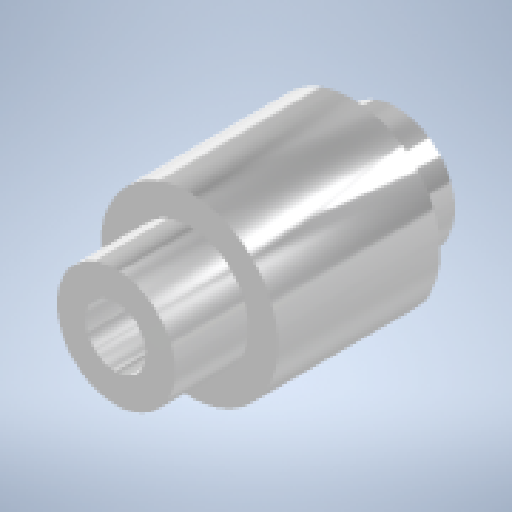
# Autodesk Inventor part: ベース板連結棒
Saved by Autodesk Inventor 2024 (Build 280153000, 153)
## iProperties
Created: 2023-05-30
Part Number: ベース板連結棒
Material: アルミニウム 6061
Document SubType Name: Modeling
Designer: yuta2
Density: 2.7 g/cm^3
Appearance: アルミニウム - フラット
Author: yuta2
Autodesk Inventor part; units mm, degrees
ref_plane "YZ Plane" through (0, 0, 0) normal (1, 0, 0) x (0, 1, 0)
ref_plane "XZ Plane" through (0, 0, 0) normal (0, 1, 0) x (-1, 0, 0)
ref_plane "XY Plane" through (0, 0, 0) normal (0, 0, 1) x (1, 0, 0)
sketch "スケッチ1" plane through (0, 0, 0) normal (1, 0, 0) x (0, 1, 0)
  line L0 (0, 0) -> (4, 0)
  line L1 (4, 0) -> (4, 5)
  line L2 (4, 5) -> (0, 5)
  line L3 (0, 5) -> (0, 0)
  line L4 (0, 0) -> (6, 0)
  line L5 (6, 0) -> (6, -11)
  line L6 (6, -11) -> (0, -11)
  line L7 (0, -11) -> (0, 0)
  line L8 (0, -11) -> (4, -11)
  line L9 (4, -11) -> (4, -14)
  line L10 (4, -14) -> (0, -14)
  line L11 (0, -14) -> (0, -11)
  dimension "d0" = 4
  dimension "d1" = 5
  dimension "d2" = 6
  dimension "d3" = 11
  dimension "d4" = 4
  dimension "d5" = 3
  constraints: 24 end point, 6 parallel, 3 horizontal, 3 perpendicular
  measures "d0" distance of L2.end L1.end
  measures "d1" distance of L1.end L0.end
  measures "d2" distance of L5.end L6.end
  measures "d3" distance of L4.end L5.end
  measures "d4" distance of L9.end L10.end
  measures "d5" distance of L8.end L9.end
revolve "回転1" add sketch "スケッチ1" angle 360 about axis through (0, 0, -11) along (0, 0, 1)
sketch "スケッチ2" plane through (0, 0, 5) normal (0, 0, 1) x (1, 0, 0)
  point P0 (0, 0)
  point P1 (0, 0)
  constraints: 1 coincident
hole "穴1" at (0, 0, 5) direction (0, 0, -1) diameter 4.1 end through all
